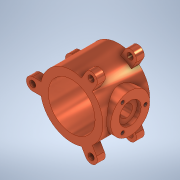
# Autodesk Inventor part: Corpo da Valvula
Saved by Autodesk Inventor 2021 (Build 250183000, 183)
## iProperties
Created: 2021-04-08
Part Number: Corpo da Valvula
Material: Genérico
Document SubType Name: Modeling
Designer: rubia
Density: 1 g/cm^3
Appearance: Metal quente 1400F
Author: rubia
Autodesk Inventor part; units mm, degrees
ref_plane "XZ Plane" through (0, 0, 0) normal (0, 1, 0) x (-1, 0, 0)
sketch "Esboço1" plane through (0, 0, 0) normal (0, 0, 1) x (1, 0, 0)
  circle A0 centre (0, 0) radius 30
  circle A1 centre (0, 0) radius 40
  dimension "d0" = 60
  dimension "d1" = 80
  constraints: 2 centre point, 2 coincident
  measures "d0" diameter of A0
  measures "d1" diameter of A1
extrude "Extrusão1" add sketch "Esboço1" along normal blind 60
sketch "Esboço2" plane through (0, 0, 60) normal (0, 0, 1) x (1, 0, 0)
  circle A0 centre (-50, 0) radius 4
  arc A1 (-50, 8) -> (-50, -8) centre (-50, 0) ccw
  line L0 (-50, 8) -> (-39.1918, 8)
  circle A2 centre (0, 0) radius 40 projected
  line L1 (-50, -8) -> (-39.1918, -8)
  arc A3 (-39.1918, 8) -> (-39.1918, -8) centre (0, 0) ccw
  dimension "d4" = 8
  dimension "d5" = 16
  dimension "d6" = 50
  constraints: 6 point on circle, 4 end point, 3 centre point, 2 coincident, 1 horizontal, 1 parallel
  measures "d4" diameter of A0
  measures "d5" diameter of A1
  measures "d6" distance of point (0, 0) A0.centre
extrude "Extrusão2" add sketch "Esboço2" against normal blind 10 contours L0 A2 L1 A1
pattern_circular "Padrão circular1" count 3 over 360 about axis through (0, 0, 0) along (0, 0, 1) of "Extrusão2"
ref_plane "Plano de trabalho1" through (0, 0, 30) normal (0, 0, 1) x (1, 0, 0)
mirror "Espelhamento1" about plane through (0, 0, 30) normal (0, 0, 1) of "Extrusão2", "Padrão circular1", "Extrusão1"
ref_plane "Plano de trabalho2" through (40, 0, 0) normal (1, 0, 0) x (0, 1, 0)
sketch "Esboço3" plane through (40, 0, 0) normal (1, 0, 0) x (0, 1, 0)
  line L0 (0, 0) -> (0, 60) construction
  line L1 (-4, 60) -> (4, 60) construction
  circle A0 centre (0, 30) radius 25
  dimension "d14" = 50
  constraints: 2 end point, 2 midpoint, 1 centre point
  measures "d14" diameter of A0
extrude "Extrusão3" add sketch "Esboço3" along normal blind 5 and the other way blind 10
sketch "Esboço4" plane through (45, 0, 30) normal (1, 0, 0) x (0, 0, -1)
  circle A0 centre (0, 0) radius 8
  point P0 (30, 0)
  dimension "d19" = 16
  constraints: 1 centre point
  measures "d19" diameter of A0
extrude "Extrusão4" cut sketch "Esboço4" against normal up to next
sketch "Esboço5" plane through (45, 0, 30) normal (1, 0, 0) x (0, 0, -1)
  circle A0 centre (0, 0) radius 14
  circle A1 centre (0, 0) radius 8
  point P0 (30, 0)
  dimension "d22" = 28
  dimension "d23" = 16
  constraints: 2 centre point, 1 coincident
  measures "d22" diameter of A0
  measures "d23" diameter of A1
extrude "Extrusão5" cut sketch "Esboço5" against normal blind 5
sketch "Esboço6" plane through (45, 0, 30) normal (1, 0, 0) x (0, 0, -1)
  circle A0 centre (0, 0) radius 14 construction
  line L0 (14, 0) -> (25, 0) construction
  circle A1 centre (0, 0) radius 25 construction
  circle A2 centre (19.5, 0) radius 2.25
  point P0 (30, 0)
  dimension "d26" = 4.5
  constraints: 2 end point, 2 horizontal alignment, 1 centre point, 1 horizontal, 1 midpoint, 2 other
  measures "d26" diameter of A2
extrude "Extrusão6" cut sketch "Esboço6" against normal blind 10
pattern_circular "Padrão circular2" count 3 over 360 about axis through (45, 0, 30) along (-1, 0, 0) of "Extrusão6"
thread "Rosca1" size "M4.5x0.5" class "6H" standard "ANSI Metric M Profile" length 3
thread "Rosca2" size "M4.5x0.5" class "6H" standard "ANSI Metric M Profile" length 3
thread "Rosca3" size "M4.5x0.5" class "6H" standard "ANSI Metric M Profile" length 3
